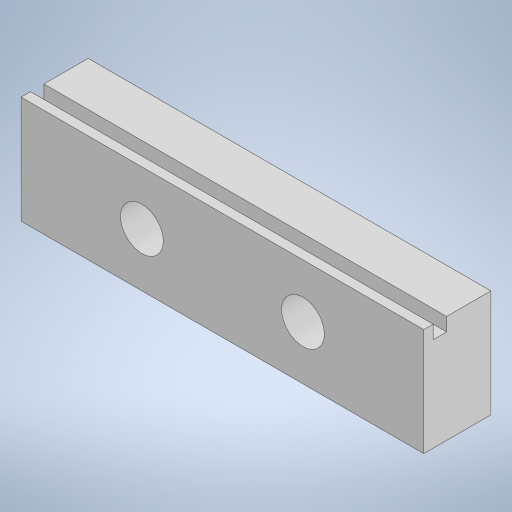
# Autodesk Inventor part: cutter_stopper
Saved by Autodesk Inventor 2024 (Build 280153000, 153)
## iProperties
Created: 2025-06-02
Part Number: cutter_stopper
Material: 一般
Document SubType Name: Modeling
Designer: 1412z
Density: 1 g/cm^3
Appearance: 既定
Author: 1412z
Autodesk Inventor part; units mm, degrees
ref_plane "YZ Plane" through (0, 0, 0) normal (1, 0, 0) x (0, 1, 0)
ref_plane "XZ Plane" through (0, 0, 0) normal (0, 1, 0) x (-1, 0, 0)
ref_plane "XY Plane" through (0, 0, 0) normal (0, 0, 1) x (1, 0, 0)
sketch "スケッチ1" plane through (0, 0, 0) normal (0, 0, 1) x (1, 0, 0)
  line L0 (7.5, -2) -> (-7.5, -2)
  line L1 (-7.5, -2) -> (-7.5, 2)
  line L2 (-7.5, 2) -> (7.5, 2)
  line L3 (7.5, 2) -> (7.5, -2)
  line L4 (7.5, -2) -> (-7.5, 2) construction
  line L5 (-7.5, -2) -> (7.5, 2) construction
  point P0 (0, 0)
  dimension "d0" = 15
  dimension "d1" = 4
  constraints: 12 end point, 2 midpoint, 2 parallel, 1 horizontal, 1 perpendicular
  measures "d0" distance of L1.end L2.end
  measures "d1" distance of L0.end L1.end
extrude "押し出し1" add sketch "スケッチ1" along normal blind 2.5
sketch "スケッチ2" plane through (-7.5, 2, 0) normal (0, 1, 0) x (1, 0, 0)
  line L0 (0, -1.9) -> (15, -1.9)
  line L1 (15, 0) -> (15, -2.5) projected
  line L2 (15, -1.9) -> (15, -1.65)
  line L3 (15, -1.65) -> (0, -1.65)
  line L4 (0, -1.65) -> (0, -2.15)
  line L5 (0, -2.15) -> (15, -2.15)
  line L6 (15, -2.15) -> (15, -1.9)
  point P0 (7.5, 0)
  dimension "d4" = 0.25
  dimension "d5" = 0.5
  constraints: 12 end point, 3 point on line, 2 perpendicular, 1 collinear, 1 horizontal, 1 parallel
  measures "d4" distance of L0.end L2.end
  measures "d5" distance of L3.end L4.end
extrude "押し出し2" cut sketch "スケッチ2" against normal blind 0.5
sketch "スケッチ3" plane through (0, 0, 0) normal (0, 0, -1) x (-1, 0, 0)
  circle A0 centre (3, 0) radius 0.8
  circle A1 centre (-3, 0) radius 0.8
  point P0 (0, 0)
  dimension "d8" = 1.6
  dimension "d9" = 1.6
  constraints: 2 centre point
  measures "d8" diameter of A0
  measures "d9" diameter of A1
extrude "押し出し3" cut sketch "スケッチ3" against normal blind 5
